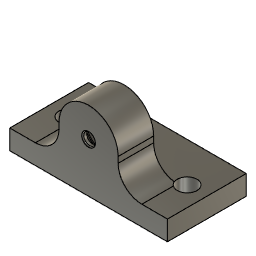
Bowden Mount (Autodesk Fusion 360 design; units mm, degrees)
Autodesk Fusion 360 part; units mm, degrees
sketch "Sketch1" plane through (0, 0, 0) normal (0, 0, 1) x (1, 0, 0)
  line L0 (20, -10) -> (-20, -10)
  line L1 (-20, -10) -> (-20, 10)
  line L2 (-20, 10) -> (20, 10)
  line L3 (20, 10) -> (20, -10)
  line L4 (20, -10) -> (-20, 10) construction
  line L5 (-20, -10) -> (20, 10) construction
  circle A0 centre (-15, 0) radius 2.5
  circle A1 centre (15, 0) radius 2.5
  dimension "d1" = 40
  dimension "d2" = 20
  dimension "d3" = 5
  dimension "d4" = 5
  dimension "d5" = 5
  dimension "d6" = 5
  dimension "d7" = 10
  dimension "d8" = 10
  constraint horizontal L0
  constraint perpendicular L0 L1
  constraint parallel L0 L2
  constraint parallel L1 L3
  constraint coincident L4 origin
  constraint coincident L5 origin
  measures "d1" distance of L1.end L2.end
  measures "d2" distance of L0.end L1.end
  measures "d3" diameter of A0
  measures "d4" diameter of A1
  measures "d5" distance of L1 A0.centre
  measures "d6" distance of L3 A1.centre
  measures "d7" distance of L2 A0.centre
  measures "d8" distance of L2 A1.centre
extrude "Extrude1" add sketch "Sketch1" along normal blind 5
sketch "Sketch2" plane through (0, 0, 5) normal (0, 0, 1) x (-1, 0, 0)
  circle A0 centre (-15, 0) radius 2.5
  circle A1 centre (15, 0) radius 2.5
  line L0 (-20, -10) -> (20, -10)
  line L1 (20, -10) -> (20, 10)
  line L2 (20, 10) -> (-20, 10)
  line L3 (-20, 10) -> (-20, -10)
  line L4 (-7.5, 5) -> (7.5, 5)
  line L5 (7.5, 5) -> (7.5, -5)
  line L6 (7.5, -5) -> (-7.5, -5)
  line L7 (-7.5, -5) -> (-7.5, 5)
  line L8 (-7.5, 5) -> (7.5, -5) construction
  line L9 (7.5, 5) -> (-7.5, -5) construction
  dimension "d11" = 15
  dimension "d12" = 10
  constraint horizontal L4
  constraint perpendicular L4 L5
  constraint parallel L4 L6
  constraint parallel L5 L7
  constraint coincident L8 origin
  constraint coincident L9 origin
  measures "d11" distance of L5.end L6.end
  measures "d12" distance of L4.end L5.end
extrude "Extrude2" add sketch "Sketch2" along normal blind 15 contours L4 L5 L6 L7
sketch "Sketch3" plane through (0, -5, 0) normal (0, -1, 0) x (1, 0, 0)
  line L0 (-7.5, 5) -> (7.5, 5)
  line L1 (7.5, 5) -> (7.5, 20)
  line L2 (7.5, 20) -> (-7.5, 20)
  line L3 (-7.5, 20) -> (-7.5, 5)
  circle A0 centre (0, 12.5) radius 4.5
  dimension "d15" = 9
  dimension "d16" = 7.5
  measures "d15" diameter of A0
  measures "d16" distance of L2 A0.centre
extrude "Extrude3" cut sketch "Sketch3" against normal blind 14 contours A0
extrude "Extrude4" add 1 faces at (0.1121, -5, 6.0042) along direction (0, -1, 0) blind 5
extrude "Extrude5" cut 1 faces at (-0.1121, 5, 18.9958) along direction (0, -1, 0) blind 6
sketch "Sketch4" plane through (0, -10, 0) normal (0, -1, 0) x (1, 0, 0)
  circle A0 centre (0, 12.5) radius 4.5
  line L0 (-20, 0) -> (20, 0)
  line L1 (20, 0) -> (20, 5)
  line L2 (20, 5) -> (7.5, 5)
  line L3 (7.5, 5) -> (7.5, 20)
  line L4 (7.5, 20) -> (-7.5, 20)
  line L5 (-7.5, 20) -> (-7.5, 5)
  line L6 (-7.5, 5) -> (-20, 5)
  line L7 (-20, 5) -> (-20, 0)
  circle A1 centre (0, 12.5) radius 1.5
  dimension "d29" = 3
  constraint concentric A0 A1
  measures "d29" diameter of A1
extrude "Extrude6" add sketch "Sketch4" against normal blind 1 contours A0
thread "Thread1" "ISO Metric profile 10.0 M10x1 6H" major diameter 10.1472 minor diameter 9.0355 pitch 1 angle 60 modelled right hand crest width 0.2748 on face at (4.4776, -7.6667, 12.0519) crest through (4.5178, -9.75, 12.5) on face at (4.4776, -2.3333, 12.0519) crest through (4.5178, -9.75, 12.5)
fillet "Fillet2" radius 7.5 2 edges at (-7.5, -2.5, 20) (7.5, -2.5, 20)
fillet "Fillet4" radius 6 2 edges at (-7.5, -5.5, 5) (7.5, -5.5, 5)
fillet "Fillet5" radius 0.25 1 edges at (-1.3985, -10, 13.0424)
equation "d6 = d5"
equation "d8 = d7"
